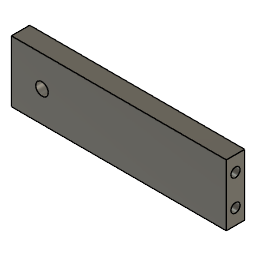
実験台2 v2 (Autodesk Fusion 360 design; units mm, degrees)
Autodesk Fusion 360 part; units mm, degrees
sketch "スケッチ1" plane through (0, 0, 0) normal (0, 0, 1) x (1, 0, 0)
  line L0 (0, 0) -> (-70, 0)
  line L1 (-70, 0) -> (-70, -6)
  line L2 (-70, -6) -> (0, -6)
  line L3 (0, -6) -> (0, 0)
  constraint horizontal L0
  constraint vertical L1
  constraint horizontal L2
  constraint vertical L3
  constraint coincident L0.start L3.end
extrude "押し出し1" add sketch "スケッチ1" along normal blind 20
sketch "スケッチ2" plane through (0, -6, 0) normal (0, -1, 0) x (1, 0, 0)
  line L0 (-70, 0) -> (0, 0)
  line L1 (0, 0) -> (0, 20)
  line L2 (0, 20) -> (-70, 20)
  line L3 (-70, 20) -> (-70, 0)
  circle A0 centre (-60, 10) radius 2.05
extrude "押し出し2" cut sketch "スケッチ2" against normal blind 6 contours A0
sketch "スケッチ3" plane through (0, 0, 0) normal (1, 0, 0) x (0, 1, 0)
  line L0 (-6, 0) -> (0, 0)
  line L1 (0, 0) -> (0, 20)
  line L2 (0, 20) -> (-6, 20)
  line L3 (-6, 20) -> (-6, 0)
  circle A0 centre (-3, 5) radius 1.5
  circle A1 centre (-3, 15) radius 1.5
extrude "押し出し3" cut sketch "スケッチ3" against normal blind 6 contours A0 | A1
